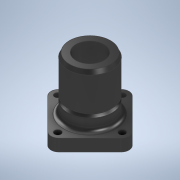
# Autodesk Inventor part: 22M_Diffuser_Port_Sq_White
Saved by Autodesk Inventor 2020 (Build 240168000, 168)
## iProperties
Created: 2021-05-14
Part Number: 22M_Diffuser_Port_Sq_White
Material: Generic
Document SubType Name: Modeling
Designer: Workshop
Density: 1 g/cm^3
Appearance: Glossy - Black
Author: Workshop
Autodesk Inventor part; units mm, degrees
ref_plane "YZ Plane" through (0, 0, 0) normal (1, 0, 0) x (0, 1, 0)
ref_plane "XZ Plane" through (0, 0, 0) normal (0, 1, 0) x (-1, 0, 0)
ref_plane "XY Plane" through (0, 0, 0) normal (0, 0, 1) x (1, 0, 0)
sketch "Sketch1" plane through (0, 0, 0) normal (0, 0, 1) x (1, 0, 0)
  line L0 (0, 7) -> (28.6, 7)
  line L1 (28.6, 7) -> (32.6, 10)
  line L2 (32.6, 10) -> (32.6, 20)
  line L3 (32.6, 20) -> (26.6, 20)
  line L4 (26.6, 20) -> (26.6, 11.125)
  line L5 (26.6, 11.125) -> (20.6, 11.125)
  line L6 (20.6, 11.125) -> (19.6, 10.125)
  line L7 (19.6, 10.125) -> (18.6, 11.125)
  line L8 (18.6, 11.125) -> (2, 11.125)
  line L9 (2, 11.125) -> (0, 10.25)
  line L10 (0, 10.25) -> (0, 7)
  line L11 (-6.52, 0) -> (39.12, 0) projected
  point P0 (0, 0)
  dimension "d2" = 3
  dimension "d3" = 4
  dimension "d4" = 6
  dimension "d5" = 6
  dimension "d6" = 20
  dimension "d7" = 4.125
  dimension "d8" = 3.25
  dimension "d9" = 2
  dimension "d10" = 2
  dimension "d11" = 1
  dimension "d12" = 1
  dimension "d13" = 7
  dimension "d26" = 32.6
  constraints: 22 end point, 4 perpendicular, 1 horizontal, 1 horizontal alignment, 1 vertical, 1 vertical alignment
  measures "d2" vertical distance of L1.end L0.end
  measures "d3" horizontal distance of L1.end L0.end
  measures "d4" distance of L2.end L3.end
  measures "d5" distance of L4.end L5.end
  measures "d6" distance from line of point (0, 0) L3
  measures "d7" distance between parallel lines of L0 L8
  measures "d8" distance of L9.end L0.start
  measures "d9" horizontal distance of L8.end L9.end
  measures "d10" distance of L5.end L7.end
  measures "d11" horizontal distance of L5.end L6.end
  measures "d12" horizontal distance of L5.end L6.end
  measures "d13" distance from line of point (0, 0) L0
  measures "d26" distance between parallel lines of L2 L10
revolve "Revolution1" add sketch "Sketch1" angle 360 about axis through (-10, 0, 0) along (1, 0, 0)
sketch "Sketch2" plane through (32.6, 0, 0) normal (1, 0, 0) x (0, 0, -1)
  circle A0 centre (0, 0) radius 20 projected
  circle A1 centre (0, 0) radius 10 projected
  circle A2 centre (-16.125, 0) radius 1.6
  circle A3 centre (0, -16.125) radius 1.6
  circle A4 centre (16.125, 0) radius 1.6
  circle A5 centre (0, 16.125) radius 1.6
  line L0 (2.8284, 18.3141) -> (18.3141, 2.8284)
  line L1 (18.3141, -2.8284) -> (2.8284, -18.3141)
  line L2 (-2.8284, -18.3141) -> (-18.3141, -2.8284)
  line L3 (-18.3141, 2.8284) -> (-2.8284, 18.3141)
  arc A6 (18.3141, -2.8284) -> (18.3141, 2.8284) centre (15.4856, 0) ccw
  arc A7 (-2.8284, -18.3141) -> (2.8284, -18.3141) centre (0, -15.4856) ccw
  arc A8 (-18.3141, 2.8284) -> (-18.3141, -2.8284) centre (-15.4856, 0) ccw
  arc A9 (2.8284, 18.3141) -> (-2.8284, 18.3141) centre (0, 15.4856) ccw
  point P0 (0, 21.1425)
  point P1 (21.1425, 0)
  point P2 (0, -21.1425)
  point P3 (-21.1425, 0)
  dimension "d15" = 3.2
  dimension "d16" = 16.125
  dimension "d19" = 360
  dimension "d21" = 29.9
  dimension "d22" = 4
  constraints: 8 centre point, 8 end point, 8 point on circle, 8 point on line, 8 tangent, 3 equal radius, 3 horizontal alignment, 2 parallel, 2 vertical alignment, 1 perpendicular, 9 other
  measures "d15" diameter of A2
  measures "d16" distance of A2.centre point (0, 0)
  measures "d21" distance of point (0, 21.142) point (21.142, 0)
  measures "d22" radius of A6
extrude "Extrusion1" cut sketch "Sketch2" against normal through all contours A0 | A2 | A3 | A4 | A5
fillet "Fillet1" radius 2 1 edges at (26.6, -11.125, 0)
body "Solid1"
